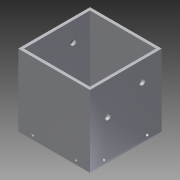
# Autodesk Inventor part: 06
Saved by Autodesk Inventor 2013 (Build 170138000, 138)
## iProperties
Created: 2014-02-01
Material: アルミニウム 6061
Document SubType Name: Modeling
Designer: andou
Density: 1 g/cm^3
Mass: 16.8573 g
Surface Area: 190.608 cm^2
Volume: 16.8573 cm^3
Part Number: 06
Author: andou
Title: Parallel_Case
Autodesk Inventor part; units mm, degrees
ref_plane "YZ Plane" through (0, 0, 0) normal (1, 0, 0) x (0, 1, 0)
ref_plane "XZ Plane" through (0, 0, 0) normal (0, 1, 0) x (-1, 0, 0)
ref_plane "XY Plane" through (0, 0, 0) normal (0, 0, 1) x (1, 0, 0)
sketch "スケッチ1" plane through (0, 0, 0) normal (0, 0, 1) x (1, 0, 0)
  line L0 (-25, 25) -> (25, 25)
  line L1 (25, 25) -> (25, -25)
  line L2 (25, -25) -> (-25, -25)
  line L3 (-25, -25) -> (-25, 25)
  line L4 (-23, 23) -> (23, 23)
  line L5 (23, 23) -> (23, -23)
  line L6 (23, -23) -> (-23, -23)
  line L7 (-23, -23) -> (-23, 23)
  point P0 (0, 0)
  dimension "d0" = 50
  dimension "d1" = 50
  dimension "d4" = 25
  dimension "d5" = 25
  dimension "d6" = 46
  dimension "d7" = 2
  dimension "d8" = 46
  dimension "d9" = 2
  constraints: 16 end point, 4 parallel, 2 horizontal, 2 perpendicular
  measures "d0" distance of L0.start L0.end
  measures "d1" distance of L2.end L0.start
  measures "d4" distance from line of L0 point (0, 0)
  measures "d5" distance from line of L3 point (0, 0)
  measures "d6" distance between parallel lines of L5 L7
  measures "d7" distance between parallel lines of L3 L7
  measures "d8" distance between parallel lines of L4 L6
  measures "d9" distance between parallel lines of L2 L6
extrude "押し出し1" add sketch "スケッチ1" along normal blind 50
sketch "スケッチ11" plane through (25, -25, 0) normal (1, 0, 0) x (0, 0, -1)
  circle A0 centre (-36.5, 36.5) radius 1.5
  line L0 (-50, 50) -> (-50, 0) projected
  circle A1 centre (-27.5, 12.5) radius 1.5
  line L1 (0, 50) -> (0, 0) projected
  line L2 (0, 50) -> (-50, 50) projected
  point P0 (0, 25)
  point P1 (-50, 43)
  dimension "d109" = 3
  dimension "d128" = 24
  dimension "d237" = 13.5
  dimension "d238" = 27.5
  dimension "d239" = 13.5
  constraints: 2 centre point, 1 equal radius
  measures "d109" diameter of A0
  measures "d128" vertical distance of A1.centre A0.centre
  measures "d237" distance from line of L2 A0.centre
  measures "d238" distance from line of L1 A1.centre
  measures "d239" distance from line of L0 A0.centre
hole "穴6" at (25, -12.5, 27.5) at (25, 11.5, 36.5) direction (-1, 0, 0) diameter 4 end through all
sketch "スケッチ16" plane through (-25, -25, 0) normal (-1, 0, 0) x (0, 0, 1)
  line L0 (0, 50) -> (50, 50) projected
  circle A0 centre (3, 40) radius 1
  circle A1 centre (3, 10) radius 1
  line L1 (0, 48) -> (0, 2) projected
  line L2 (0, 0) -> (50, 0) projected
  point P0 (0, 25)
  dimension "d175" = 10
  dimension "d176" = 3
  dimension "d178" = 3
  dimension "d287" = 10
  dimension "d288" = 2
  constraints: 2 centre point, 1 equal radius
  measures "d175" distance from line of L0 A0.centre
  measures "d176" distance from line of L1 A0.centre
  measures "d178" distance from line of L1 A1.centre
  measures "d287" distance from line of A1.centre L2
  measures "d288" diameter of A0
hole "穴16" at (-25, 15, 3) at (-25, -15, 3) direction (1, 0, 0) diameter 2 end through all
sketch "スケッチ15" plane through (-25, -25, 0) normal (0, -1, 0) x (1, 0, 0)
  line L0 (0, 0) -> (0, 50) projected
  line L1 (50, 0) -> (0, 0) projected
  circle A0 centre (10, 3) radius 1
  circle A1 centre (40, 3) radius 1
  line L2 (50, 0) -> (50, 50) projected
  point P0 (49.5, 0)
  point P1 (49.5, 50)
  point P2 (25, 0)
  dimension "d167" = 10
  dimension "d170" = 3
  dimension "d172" = 3
  dimension "d267" = 2
  dimension "d286" = 10
  constraints: 2 centre point, 1 equal radius
  measures "d167" distance from line of L0 A0.centre
  measures "d170" distance from line of L1 A0.centre
  measures "d172" distance from line of A1.centre L1
  measures "d267" diameter of A1
  measures "d286" distance from line of L2 A1.centre
hole "穴17" at (-15, -25, 3) at (15, -25, 3) direction (0, 1, 0) diameter 2 end through all
